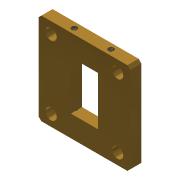
# Autodesk Inventor part: WG18FLANGE
Saved by Autodesk Inventor 2015 (Build 190159000, 159)
## iProperties
Created: 2014-03-25
Part Number: WG18FLANGE
Material: Brass, Soft Yellow
Document SubType Name: Modeling
Designer: jad211
Density: 8.47 g/cm^3
Appearance: Brass - Satin
Author: jad211
Autodesk Inventor part; units mm, degrees
ref_plane "YZ Plane" through (0, 0, 0) normal (1, 0, 0) x (0, 1, 0)
ref_plane "XZ Plane" through (0, 0, 0) normal (0, 1, 0) x (-1, 0, 0)
ref_plane "XY Plane" through (0, 0, 0) normal (0, 0, 1) x (1, 0, 0)
sketch "Sketch3" plane through (0, 0, 0) normal (0, 0, 1) x (1, 0, 0)
  line L0 (-15.7, -16.7) -> (15.7, -16.7)
  line L1 (16.7, -15.7) -> (16.7, 15.7)
  line L2 (15.7, 16.7) -> (-15.7, 16.7)
  line L3 (-16.7, 15.7) -> (-16.7, -15.7)
  line L4 (-16.7, -16.7) -> (16.7, 16.7) construction
  line L5 (16.7, -16.7) -> (-16.7, 16.7) construction
  line L6 (-15.7, 16.7) -> (-16.7, 15.7)
  line L7 (15.7, 16.7) -> (16.7, 15.7)
  line L8 (16.7, -15.7) -> (15.7, -16.7)
  line L9 (-16.7, -15.7) -> (-15.7, -16.7)
  line L10 (-4.9497, -8.8994) -> (4.9497, -8.8994)
  line L11 (4.9497, -8.8994) -> (4.9497, 8.8994)
  line L12 (4.9497, 8.8994) -> (-4.9497, 8.8994)
  line L13 (-4.9497, 8.8994) -> (-4.9497, -8.8994)
  line L14 (-4.9497, -8.8994) -> (4.9497, 8.8994) construction
  line L15 (4.9497, -8.8994) -> (-4.9497, 8.8994) construction
  circle A0 centre (-12.14, 12.625) radius 2.045
  circle A1 centre (12.14, 12.625) radius 2.045
  line L16 (0, -16.7) -> (0, 16.7) construction
  circle A2 centre (-12.14, -12.625) radius 2.045
  circle A3 centre (12.14, -12.625) radius 2.045
  line L17 (12.14, 12.625) -> (-12.14, 12.625) construction
  line L18 (-12.14, 12.625) -> (-12.14, -12.625) construction
  line L19 (-12.14, -12.625) -> (12.14, -12.625) construction
  line L20 (12.14, -12.625) -> (12.14, 12.625) construction
  line L21 (-16.7, 0) -> (16.7, 0) construction
  point P0 (0, 0)
  point P1 (0, 0)
  dimension "d0" = 33.4
  dimension "d1" = 33.4
  dimension "d2" = 1
  dimension "d3" = 1
  dimension "d4" = 1
  dimension "d5" = 1
  dimension "d6" = 1
  dimension "d7" = 1
  dimension "d8" = 1
  dimension "d9" = 1
  dimension "d10" = 9.8994
  dimension "d11" = 17.7988
  dimension "d12" = 4.09
  dimension "d13" = 4.09
  dimension "d17" = 4.09
  dimension "d19" = 24.28
  dimension "d20" = 25.25
  dimension "d21" = 4.09
  dimension "d22" = 12.625
  dimension "d23" = 12.14
  constraints: 45 end point, 10 midpoint, 8 point on line, 6 perpendicular, 4 centre point, 4 parallel, 2 horizontal
  measures "d0" distance of L5.end L4.end
  measures "d1" distance of L4.end L5.start
  measures "d2" distance of L2.end L5.end
  measures "d3" distance of L3.start L5.end
  measures "d4" distance of L2.start L4.end
  measures "d5" distance of L1.end L4.end
  measures "d6" distance of L1.start L5.start
  measures "d7" distance of L0.end L5.start
  measures "d8" distance of L3.end L4.start
  measures "d9" distance of L0.start L4.start
  measures "d10" distance of L12.end L11.end
  measures "d11" distance of L11.end L10.end
  measures "d12" diameter of A0
  measures "d13" diameter of A1
  measures "d17" diameter of A2
  measures "d19" distance of L17.start L17.end
  measures "d20" distance of L18.end L17.end
  measures "d21" diameter of A3
  measures "d22" distance from line of L21.start L17
  measures "d23" distance from line of L16 L17.start
extrude "Extrusion1" add sketch "Sketch3" along normal blind 4.1
sketch "Sketch6" plane through (-15.7, 16.7, 0) normal (0, 1, 0) x (1, 0, 0)
  circle A0 centre (10, -2.05) radius 1
  circle A1 centre (23.4, -2.05) radius 1
  line L0 (-1, 0) -> (-1, -4.1) projected
  line L1 (32.4, 0) -> (32.4, -4.1) projected
  line L2 (31.4, 0) -> (0, 0) projected
  line L3 (31.4, -4.1) -> (0, -4.1) projected
  point P0 (15.7, 0)
  dimension "d54" = 2
  dimension "d55" = 2
  dimension "d57" = 9
  dimension "d58" = 13.4
  dimension "d59" = 2.05
  dimension "d60" = 2.05
  constraints: 2 centre point
  measures "d54" diameter of A0
  measures "d55" diameter of A1
  measures "d57" distance from line of A1.centre L1
  measures "d58" distance of A1.centre A0.centre
  measures "d59" distance from line of L2 A0.centre
  measures "d60" distance from line of A0.centre L3
sketch "Sketch7" plane through (-15.7, -16.7, 0) normal (0, -1, 0) x (1, 0, 0)
  circle A0 centre (23.4, 2.05) radius 1
  circle A1 centre (10, 2.05) radius 1
  line L0 (0, 0) -> (31.4, 0) projected
  line L1 (0, 4.1) -> (31.4, 4.1) projected
  line L2 (32.4, 0) -> (32.4, 4.1) projected
  line L3 (-1, 0) -> (-1, 4.1) projected
  point P0 (15.7, 0)
  dimension "d61" = 2
  dimension "d62" = 2
  dimension "d63" = 2.05
  dimension "d64" = 2.05
  dimension "d65" = 2.05
  dimension "d67" = 11
  dimension "d81" = 13.4
  constraints: 2 centre point
  measures "d61" diameter of A0
  measures "d62" diameter of A1
  measures "d63" distance from line of L0 A0.centre
  measures "d64" distance from line of L1 A0.centre
  measures "d65" distance from line of L1 A1.centre
  measures "d67" distance from line of L3 A1.centre
  measures "d81" distance of A0.centre A1.centre
extrude "Extrusion4" cut sketch "Sketch7" against normal blind 8
extrude "Extrusion5" cut sketch "Sketch6" against normal blind 7
thread "Thread5" size "M2x0.4" class "6H" standard "ANSI Metric M Profile" full length
thread "Thread6" size "M2x0.4" class "6H" standard "ANSI Metric M Profile" full length
thread "Thread7" size "M2x0.4" class "6H" standard "ANSI Metric M Profile" full length
thread "Thread8" size "M2x0.4" class "6H" standard "ANSI Metric M Profile" full length
equation "\"d3\" = d2"
equation "\"d5\" = d4"
equation "\"d6\" = d4"
equation "\"d7\" = d6"
equation "\"d8\" = d4"
equation "\"d9\" = d8"
body "Solid1"
